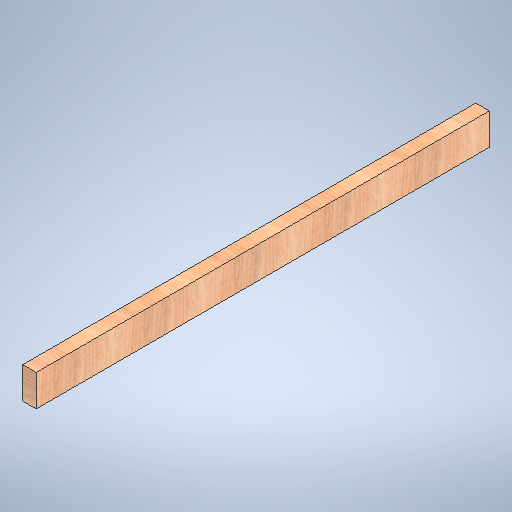
# Autodesk Inventor part: Header_With_Dimensions_1.5_x_3.5_x_50.25_Inches
Saved by Autodesk Inventor 2025 (Build 290162010, 162A)
## iProperties
Created: 2024-10-13
Part Number: Header_With_Dimensions_1.5_x_3.5_x_50.25_Inches
Material: Wood (Birch)
Document SubType Name: Modeling
Designer: Tom
Density: 0.55 g/cm^3
Appearance: Birch - Natural Polished
Author: Tom
Autodesk Inventor part; units mm, degrees
ref_plane "YZ Plane" through (0, 0, 0) normal (1, 0, 0) x (0, 1, 0)
ref_plane "XZ Plane" through (0, 0, 0) normal (0, 1, 0) x (-1, 0, 0)
ref_plane "XY Plane" through (0, 0, 0) normal (0, 0, 1) x (1, 0, 0)
sketch "Sketch1" plane through (0, 0, 0) normal (1, 0, 0) x (0, 1, 0)
  line L0 (0, 0) -> (88.9, 0)
  line L1 (88.9, 0) -> (88.9, -1276.35)
  line L2 (88.9, -1276.35) -> (0, -1276.35)
  line L3 (0, -1276.35) -> (0, 0)
  dimension "d1" = 1276.35
  dimension "d4" = 88.9
  constraints: 8 end point, 2 parallel, 1 horizontal, 1 perpendicular
  measures "d1" distance of L2.end L0.start
  measures "d4" distance of L0.start L0.end
extrude "Extrusion1" add sketch "Sketch1" along normal blind 38.1
body "Solid1"
